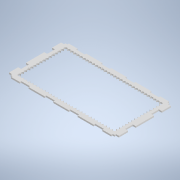
# Autodesk Inventor part: 2x pcb board holer
Saved by Autodesk Inventor 2022 (Build 260153000, 153)
## iProperties
Created: 2021-06-29
Part Number: 2x pcb board holer
Material: Generic
Document SubType Name: Modeling
Designer: benka
Density: 1 g/cm^3
Appearance: Default
Author: benka
Autodesk Inventor part; units mm, degrees
ref_plane "YZ Plane" through (0, 0, 0) normal (1, 0, 0) x (0, 1, 0)
ref_plane "XZ Plane" through (0, 0, 0) normal (0, 1, 0) x (-1, 0, 0)
ref_plane "XY Plane" through (0, 0, 0) normal (0, 0, 1) x (1, 0, 0)
sketch "Sketch1" plane through (-0.0872, 0, 0.1488) normal (0, 1, 0) x (-1, 0, 0)
  line L0 (-27.5872, -94.1488) -> (-27.5872, -99.1488)
  line L1 (-27.5872, -99.1488) -> (27.4128, -99.1488)
  line L2 (27.4128, -94.1488) -> (27.4128, -99.1488)
  circle A0 centre (-42.0872, -84.1488) radius 1
  line L3 (-57.5872, -94.1488) -> (-27.5872, -94.1488)
  line L4 (-57.5872, -94.1488) -> (-57.5872, -99.1488)
  circle A1 centre (-42.0872, 83.8512) radius 1
  line L5 (-57.5872, 93.8512) -> (-57.5872, 98.8512)
  line L6 (-57.5872, 93.8512) -> (-27.5872, 93.8512)
  line L7 (-27.5872, 93.8512) -> (-27.5872, 98.8512)
  line L8 (-27.5872, 98.8512) -> (27.4128, 98.8512)
  line L9 (27.4128, 93.8512) -> (27.4128, 98.8512)
  circle A2 centre (41.9128, -84.1488) radius 1
  line L10 (93.9128, -57.8988) -> (93.9128, -31.6488)
  circle A3 centre (83.9128, -42.1488) radius 1
  line L11 (103.9128, -57.8988) -> (93.9128, -57.8988)
  line L12 (103.9128, -89.1488) -> (103.9128, -57.8988)
  line L13 (103.9128, -89.1488) -> (93.9128, -89.1488)
  line L14 (57.4128, -94.1488) -> (57.4128, -99.1488)
  line L15 (57.4128, -99.1488) -> (87.4128, -99.1488)
  line L16 (87.4128, -94.1488) -> (87.4128, -99.1488)
  line L17 (93.9128, -94.1488) -> (87.4128, -94.1488)
  line L18 (93.9128, -89.1488) -> (93.9128, -94.1488)
  line L19 (103.9128, -31.6488) -> (93.9128, -31.6488)
  line L20 (27.4128, -94.1488) -> (57.4128, -94.1488)
  line L21 (103.9128, 31.3512) -> (93.9128, 31.3512)
  line L22 (103.9128, 57.6012) -> (93.9128, 57.6012)
  line L23 (103.9128, 57.6012) -> (103.9128, 88.8512)
  line L24 (93.9128, 93.8512) -> (87.4128, 93.8512)
  line L25 (93.9128, 88.8512) -> (103.9128, 88.8512)
  line L26 (93.9128, 88.8512) -> (93.9128, 93.8512)
  line L27 (27.4128, 93.8512) -> (57.4128, 93.8512)
  circle A4 centre (41.9128, 83.8512) radius 1
  circle A5 centre (83.9128, 41.8512) radius 1
  line L28 (57.4128, 93.8512) -> (57.4128, 98.8512)
  line L29 (93.9128, 31.3512) -> (93.9128, 57.6012)
  line L30 (57.4128, 98.8512) -> (87.4128, 98.8512)
  line L31 (87.4128, 93.8512) -> (87.4128, 98.8512)
  line L32 (103.9128, -31.6488) -> (103.9128, 31.3512)
  arc A6 (-52.5872, 78.6012) -> (-63.0872, 78.6012) centre (-57.8372, 78.6012) ccw
  arc A7 (-42.0872, 78.6012) -> (-52.5872, 78.6012) centre (-47.3372, 78.6012) ccw
  arc A8 (-31.5872, 78.6012) -> (-42.0872, 78.6012) centre (-36.8372, 78.6012) ccw
  arc A9 (-21.0872, 78.6012) -> (-31.5872, 78.6012) centre (-26.3372, 78.6012) ccw
  arc A10 (-10.5872, 78.6012) -> (-21.0872, 78.6012) centre (-15.8372, 78.6012) ccw
  arc A11 (-0.0872, 78.6012) -> (-10.5872, 78.6012) centre (-5.3372, 78.6012) ccw
  arc A12 (10.4128, 78.6012) -> (-0.0872, 78.6012) centre (5.1628, 78.6012) ccw
  arc A13 (20.9128, 78.6012) -> (10.4128, 78.6012) centre (15.6628, 78.6012) ccw
  arc A14 (31.4128, 78.6012) -> (20.9128, 78.6012) centre (26.1628, 78.6012) ccw
  arc A15 (41.9128, 78.6012) -> (31.4128, 78.6012) centre (36.6628, 78.6012) ccw
  arc A16 (52.4128, 78.6012) -> (41.9128, 78.6012) centre (47.1628, 78.6012) ccw
  arc A17 (62.9128, 78.6012) -> (52.4128, 78.6012) centre (57.6628, 78.6012) ccw
  arc A18 (73.4128, 78.6012) -> (62.9128, 78.6012) centre (68.1628, 78.6012) ccw
  arc A19 (78.6628, -0.1488) -> (78.6628, 10.3512) centre (78.6628, 5.1012) ccw
  arc A20 (78.6628, 10.3512) -> (78.6628, 20.8512) centre (78.6628, 15.6012) ccw
  arc A21 (78.6628, 20.8512) -> (78.6628, 31.3512) centre (78.6628, 26.1012) ccw
  arc A22 (78.6628, 31.3512) -> (78.6628, 41.8512) centre (78.6628, 36.6012) ccw
  arc A23 (78.6628, 73.3512) -> (73.4128, 78.6012) centre (78.6628, 78.6012) ccw
  arc A24 (78.6628, 62.8512) -> (78.6628, 73.3512) centre (78.6628, 68.1012) ccw
  arc A25 (78.6628, 52.3512) -> (78.6628, 62.8512) centre (78.6628, 57.6012) ccw
  arc A26 (78.6628, 41.8512) -> (78.6628, 52.3512) centre (78.6628, 47.1012) ccw
  arc A27 (78.6628, -10.6488) -> (78.6628, -0.1488) centre (78.6628, -5.3988) ccw
  arc A28 (78.6628, -21.1488) -> (78.6628, -10.6488) centre (78.6628, -15.8988) ccw
  arc A29 (78.6628, -31.6488) -> (78.6628, -21.1488) centre (78.6628, -26.3988) ccw
  arc A30 (78.6628, -42.1488) -> (78.6628, -31.6488) centre (78.6628, -36.8988) ccw
  arc A31 (31.4128, -78.8988) -> (41.9128, -78.8988) centre (36.6628, -78.8988) ccw
  arc A32 (-10.5872, -78.8988) -> (-0.0872, -78.8988) centre (-5.3372, -78.8988) ccw
  arc A33 (-0.0872, -78.8988) -> (10.4128, -78.8988) centre (5.1628, -78.8988) ccw
  arc A34 (10.4128, -78.8988) -> (20.9128, -78.8988) centre (15.6628, -78.8988) ccw
  arc A35 (20.9128, -78.8988) -> (31.4128, -78.8988) centre (26.1628, -78.8988) ccw
  arc A36 (-63.0872, -78.8988) -> (-52.5872, -78.8988) centre (-57.8372, -78.8988) ccw
  arc A37 (-21.0872, -78.8988) -> (-10.5872, -78.8988) centre (-15.8372, -78.8988) ccw
  arc A38 (-31.5872, -78.8988) -> (-21.0872, -78.8988) centre (-26.3372, -78.8988) ccw
  arc A39 (-42.0872, -78.8988) -> (-31.5872, -78.8988) centre (-36.8372, -78.8988) ccw
  arc A40 (-52.5872, -78.8988) -> (-42.0872, -78.8988) centre (-47.3372, -78.8988) ccw
  arc A41 (41.9128, -78.8988) -> (52.4128, -78.8988) centre (47.1628, -78.8988) ccw
  arc A42 (52.4128, -78.8988) -> (62.9128, -78.8988) centre (57.6628, -78.8988) ccw
  arc A43 (62.9128, -78.8988) -> (73.4128, -78.8988) centre (68.1628, -78.8988) ccw
  arc A44 (78.6628, -52.6488) -> (78.6628, -42.1488) centre (78.6628, -47.3988) ccw
  arc A45 (78.6628, -63.1488) -> (78.6628, -52.6488) centre (78.6628, -57.8988) ccw
  arc A46 (78.6628, -73.6488) -> (78.6628, -63.1488) centre (78.6628, -68.3988) ccw
  arc A47 (73.4128, -78.8988) -> (78.6628, -73.6488) centre (78.6628, -78.8988) ccw
  arc A48 (-73.5872, -78.8988) -> (-63.0872, -78.8988) centre (-68.3372, -78.8988) ccw
  arc A49 (-63.0872, 78.6012) -> (-73.5872, 78.6012) centre (-68.3372, 78.6012) ccw
  arc A50 (-84.0872, -78.8988) -> (-73.5872, -78.8988) centre (-78.8372, -78.8988) ccw
  arc A51 (-73.5872, 78.6012) -> (-84.0872, 78.6012) centre (-78.8372, 78.6012) ccw
  line L33 (-140.5872, -94.1488) -> (-140.5872, -99.1488)
  line L34 (-140.5872, -99.1488) -> (-195.5872, -99.1488)
  line L35 (-195.5872, -94.1488) -> (-195.5872, -99.1488)
  circle A52 centre (-126.0872, -84.1488) radius 1
  line L36 (-110.5872, -94.1488) -> (-140.5872, -94.1488)
  line L37 (-110.5872, -94.1488) -> (-110.5872, -99.1488)
  circle A53 centre (-126.0872, 83.8512) radius 1
  line L38 (-110.5872, 93.8512) -> (-110.5872, 98.8512)
  line L39 (-110.5872, 93.8512) -> (-140.5872, 93.8512)
  line L40 (-140.5872, 93.8512) -> (-140.5872, 98.8512)
  line L41 (-140.5872, 98.8512) -> (-195.5872, 98.8512)
  line L42 (-195.5872, 93.8512) -> (-195.5872, 98.8512)
  circle A54 centre (-210.0872, -84.1488) radius 1
  line L43 (-262.0872, -57.8988) -> (-262.0872, -31.6488)
  circle A55 centre (-252.0872, -42.1488) radius 1
  line L44 (-272.0872, -57.8988) -> (-262.0872, -57.8988)
  line L45 (-272.0872, -89.1488) -> (-272.0872, -57.8988)
  line L46 (-272.0872, -89.1488) -> (-262.0872, -89.1488)
  line L47 (-225.5872, -94.1488) -> (-225.5872, -99.1488)
  line L48 (-225.5872, -99.1488) -> (-255.5872, -99.1488)
  line L49 (-255.5872, -94.1488) -> (-255.5872, -99.1488)
  line L50 (-262.0872, -94.1488) -> (-255.5872, -94.1488)
  line L51 (-262.0872, -89.1488) -> (-262.0872, -94.1488)
  line L52 (-272.0872, -31.6488) -> (-262.0872, -31.6488)
  line L53 (-195.5872, -94.1488) -> (-225.5872, -94.1488)
  line L54 (-272.0872, 31.3512) -> (-262.0872, 31.3512)
  line L55 (-272.0872, 57.6012) -> (-262.0872, 57.6012)
  line L56 (-272.0872, 57.6012) -> (-272.0872, 88.8512)
  line L57 (-262.0872, 93.8512) -> (-255.5872, 93.8512)
  line L58 (-262.0872, 88.8512) -> (-272.0872, 88.8512)
  line L59 (-262.0872, 88.8512) -> (-262.0872, 93.8512)
  line L60 (-195.5872, 93.8512) -> (-225.5872, 93.8512)
  circle A56 centre (-210.0872, 83.8512) radius 1
  circle A57 centre (-252.0872, 41.8512) radius 1
  line L61 (-225.5872, 93.8512) -> (-225.5872, 98.8512)
  line L62 (-262.0872, 31.3512) -> (-262.0872, 57.6012)
  line L63 (-225.5872, 98.8512) -> (-255.5872, 98.8512)
  line L64 (-255.5872, 93.8512) -> (-255.5872, 98.8512)
  line L65 (-272.0872, -31.6488) -> (-272.0872, 31.3512)
  arc A58 (-105.0872, 78.6012) -> (-115.5872, 78.6012) centre (-110.3372, 78.6012) ccw
  arc A59 (-115.5872, 78.6012) -> (-126.0872, 78.6012) centre (-120.8372, 78.6012) ccw
  arc A60 (-126.0872, 78.6012) -> (-136.5872, 78.6012) centre (-131.3372, 78.6012) ccw
  arc A61 (-136.5872, 78.6012) -> (-147.0872, 78.6012) centre (-141.8372, 78.6012) ccw
  arc A62 (-147.0872, 78.6012) -> (-157.5872, 78.6012) centre (-152.3372, 78.6012) ccw
  arc A63 (-157.5872, 78.6012) -> (-168.0872, 78.6012) centre (-162.8372, 78.6012) ccw
  arc A64 (-168.0872, 78.6012) -> (-178.5872, 78.6012) centre (-173.3372, 78.6012) ccw
  arc A65 (-178.5872, 78.6012) -> (-189.0872, 78.6012) centre (-183.8372, 78.6012) ccw
  arc A66 (-189.0872, 78.6012) -> (-199.5872, 78.6012) centre (-194.3372, 78.6012) ccw
  arc A67 (-199.5872, 78.6012) -> (-210.0872, 78.6012) centre (-204.8372, 78.6012) ccw
  arc A68 (-210.0872, 78.6012) -> (-220.5872, 78.6012) centre (-215.3372, 78.6012) ccw
  arc A69 (-220.5872, 78.6012) -> (-231.0872, 78.6012) centre (-225.8372, 78.6012) ccw
  arc A70 (-231.0872, 78.6012) -> (-241.5872, 78.6012) centre (-236.3372, 78.6012) ccw
  arc A71 (-246.8372, 10.3512) -> (-246.8372, -0.1488) centre (-246.8372, 5.1012) ccw
  arc A72 (-246.8372, 20.8512) -> (-246.8372, 10.3512) centre (-246.8372, 15.6012) ccw
  arc A73 (-246.8372, 31.3512) -> (-246.8372, 20.8512) centre (-246.8372, 26.1012) ccw
  arc A74 (-246.8372, 41.8512) -> (-246.8372, 31.3512) centre (-246.8372, 36.6012) ccw
  arc A75 (-241.5872, 78.6012) -> (-246.8372, 73.3512) centre (-246.8372, 78.6012) ccw
  arc A76 (-246.8372, 73.3512) -> (-246.8372, 62.8512) centre (-246.8372, 68.1012) ccw
  arc A77 (-246.8372, 62.8512) -> (-246.8372, 52.3512) centre (-246.8372, 57.6012) ccw
  arc A78 (-246.8372, 52.3512) -> (-246.8372, 41.8512) centre (-246.8372, 47.1012) ccw
  arc A79 (-246.8372, -0.1488) -> (-246.8372, -10.6488) centre (-246.8372, -5.3988) ccw
  arc A80 (-246.8372, -10.6488) -> (-246.8372, -21.1488) centre (-246.8372, -15.8988) ccw
  arc A81 (-246.8372, -21.1488) -> (-246.8372, -31.6488) centre (-246.8372, -26.3988) ccw
  arc A82 (-246.8372, -31.6488) -> (-246.8372, -42.1488) centre (-246.8372, -36.8988) ccw
  arc A83 (-210.0872, -78.8988) -> (-199.5872, -78.8988) centre (-204.8372, -78.8988) ccw
  arc A84 (-168.0872, -78.8988) -> (-157.5872, -78.8988) centre (-162.8372, -78.8988) ccw
  arc A85 (-178.5872, -78.8988) -> (-168.0872, -78.8988) centre (-173.3372, -78.8988) ccw
  arc A86 (-189.0872, -78.8988) -> (-178.5872, -78.8988) centre (-183.8372, -78.8988) ccw
  arc A87 (-199.5872, -78.8988) -> (-189.0872, -78.8988) centre (-194.3372, -78.8988) ccw
  arc A88 (-115.5872, -78.8988) -> (-105.0872, -78.8988) centre (-110.3372, -78.8988) ccw
  arc A89 (-157.5872, -78.8988) -> (-147.0872, -78.8988) centre (-152.3372, -78.8988) ccw
  arc A90 (-147.0872, -78.8988) -> (-136.5872, -78.8988) centre (-141.8372, -78.8988) ccw
  arc A91 (-136.5872, -78.8988) -> (-126.0872, -78.8988) centre (-131.3372, -78.8988) ccw
  arc A92 (-126.0872, -78.8988) -> (-115.5872, -78.8988) centre (-120.8372, -78.8988) ccw
  arc A93 (-220.5872, -78.8988) -> (-210.0872, -78.8988) centre (-215.3372, -78.8988) ccw
  arc A94 (-231.0872, -78.8988) -> (-220.5872, -78.8988) centre (-225.8372, -78.8988) ccw
  arc A95 (-241.5872, -78.8988) -> (-231.0872, -78.8988) centre (-236.3372, -78.8988) ccw
  arc A96 (-246.8372, -42.1488) -> (-246.8372, -52.6488) centre (-246.8372, -47.3988) ccw
  arc A97 (-246.8372, -52.6488) -> (-246.8372, -63.1488) centre (-246.8372, -57.8988) ccw
  arc A98 (-246.8372, -63.1488) -> (-246.8372, -73.6488) centre (-246.8372, -68.3988) ccw
  arc A99 (-246.8372, -73.6488) -> (-241.5872, -78.8988) centre (-246.8372, -78.8988) ccw
  arc A100 (-105.0872, -78.8988) -> (-94.5872, -78.8988) centre (-99.8372, -78.8988) ccw
  arc A101 (-94.5872, 78.6012) -> (-105.0872, 78.6012) centre (-99.8372, 78.6012) ccw
  arc A102 (-94.5872, -78.8988) -> (-84.0872, -78.8988) centre (-89.3372, -78.8988) ccw
  arc A103 (-84.0872, 78.6012) -> (-94.5872, 78.6012) centre (-89.3372, 78.6012) ccw
  line L66 (-57.5872, -99.1488) -> (-110.5872, -99.1488)
  line L67 (-110.5872, 98.8512) -> (-57.5872, 98.8512)
  point P0 (-0.0872, -0.1488)
  point P1 (-0.0001, 0)
  point P2 (-84.0872, -0.1488)
  point P3 (-168.0872, -0.1488)
  point P4 (-168.1742, 0)
  point P5 (-73.5872, -78.8988)
  point P6 (-94.5872, -78.8988)
  point P7 (-105.0872, -78.8988)
  point P8 (-105.0872, 78.6012)
  point P9 (-94.5872, 78.6012)
  point P10 (-73.5872, 78.6012)
  point P11 (-63.0872, 78.6012)
  dimension "d0" = 10
  dimension "d1" = 10.5
  dimension "d6" = 10
  dimension "d7" = 10.5
  dimension "d36" = 31.25
  dimension "d57" = 2
  dimension "d43" = 2
  dimension "d31" = 2
  dimension "d40" = 2
  dimension "d32" = 84
  dimension "d33" = 84
  dimension "d37" = 30
  dimension "d38" = 30
  dimension "d58" = 55
  dimension "d56" = 30
  dimension "d63" = 5
  dimension "d39" = 31.25
  dimension "d64" = 26.25
  dimension "d65" = 63
  dimension "d66" = 26.25
  dimension "d34" = 5
  dimension "d29" = 5
  dimension "d35" = 10
  dimension "d67" = 6.5
  dimension "d68" = 30
  dimension "d69" = 55
  dimension "d70" = 30
  dimension "d30" = 5
  dimension "d74" = 5
  dimension "d28" = 104
  dimension "d27" = 99
  dimension "d26" = 84
  dimension "d24" = 84
  dimension "d21" = 42
  dimension "d75" = 42
  dimension "d20" = 84
  dimension "d19" = 42
  dimension "d77" = 42
  dimension "d18" = 42
  dimension "d78" = 42
  dimension "d17" = 84
  dimension "d16" = 84
  dimension "d92" = 10.5
  dimension "d100" = 10.5
  dimension "d107" = 10.5
  dimension "d113" = 53
  constraints: 184 point on circle, 138 end point, 104 centre point, 29 perpendicular, 11 collinear, 4 horizontal, 1 parallel, 1 vertical, 17 other
  measures "d36" distance of L23.end L22.start
  measures "d57" diameter of A0
  measures "d43" diameter of A1
  measures "d31" diameter of A5
  measures "d40" diameter of A3
  measures "d32" distance of A3.centre A5.centre
  measures "d33" distance of A1.centre A4.centre
  measures "d37" distance between parallel lines of L14 L16
  measures "d38" distance between parallel lines of L2 L14
  measures "d58" distance between parallel lines of L0 L2
  measures "d56" distance between parallel lines of L4 L0
  measures "d63" distance between parallel lines of L17 L15
  measures "d39" distance of L12.start L11.start
  measures "d64" distance of L10.start L10.end
  measures "d65" distance of L19.start L21.start
  measures "d66" distance of L21.end L22.end
  measures "d34" distance of L25.start L24.start
  measures "d29" distance of L24.end L30.end
  measures "d35" distance of L25.start L23.end
  measures "d67" distance of L24.start L24.end
  measures "d68" distance of L28.end L30.end
  measures "d69" distance of L7.end L8.end
  measures "d70" distance of L5.start L6.end
  measures "d30" distance of L27.end L28.end
  measures "d74" distance of L9.start L8.end
  measures "d28" distance from line of L32 point (-0.087, -0.149)
  measures "d27" distance from line of L8 point (-0.087, -0.149)
  measures "d26" horizontal distance of A3.centre point (-0.087, -0.149)
  measures "d24" horizontal distance of A5.centre point (-0.087, -0.149)
  measures "d21" vertical distance of A5.centre point (-0.087, -0.149)
  measures "d75" vertical distance of A3.centre point (-0.087, -0.149)
  measures "d20" vertical distance of A0.centre point (-0.087, -0.149)
  measures "d19" horizontal distance of A2.centre point (-0.087, -0.149)
  measures "d77" horizontal distance of A0.centre point (-0.087, -0.149)
  measures "d18" horizontal distance of A4.centre point (-0.087, -0.149)
  measures "d78" horizontal distance of A1.centre point (-0.087, -0.149)
  measures "d17" vertical distance of A4.centre point (-0.087, -0.149)
  measures "d16" vertical distance of A1.centre point (-0.087, -0.149)
  measures "d92" distance of A36.centre A48.centre
  measures "d100" distance of A6.centre A49.centre
  measures "d107" distance of A48.centre A50.centre
  measures "d113" distance of L4.end L37.end
extrude "2x board holder" add sketch "Sketch1" along normal blind 5
body "Solid1"
